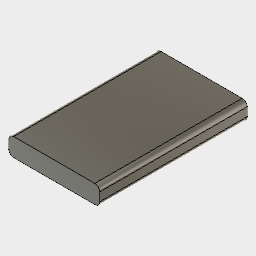
2011 2000mAh Battery (Autodesk Fusion 360 design; units mm, degrees)
Autodesk Fusion 360 part; units mm, degrees
sketch "Sketch1" plane through (0, 0, 0) normal (0, 0, 1) x (1, 0, 0)
  line L0 (18.5, -30) -> (-18.5, -30)
  line L1 (-18.5, -30) -> (-18.5, 30)
  line L2 (-18.5, 30) -> (18.5, 30)
  line L3 (18.5, 30) -> (18.5, -30)
  line L4 (18.5, -30) -> (-18.5, 30) construction
  line L5 (-18.5, -30) -> (18.5, 30) construction
  dimension "d1" = 60
  dimension "d2" = 37
  measures "d1" distance of L0.end L1.end
  measures "d2" distance of L1.end L2.end
extrude "Extrude1" add sketch "Sketch1" along normal blind 7.5
fillet "Fillet1" radius 2 4 edges at (18.5, 0, 7.5) (18.5, 0, 0) (-18.5, 0, 7.5) (-18.5, 0, 0)
